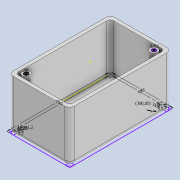
# Autodesk Inventor part: proper shit spodnji
Saved by Autodesk Inventor 2020 (Build 240168000, 168)
## iProperties
Created: 2020-08-03
Part Number: proper shit spodnji
Material: Generic
Document SubType Name: Modeling
Designer: borbu
Density: 1 g/cm^3
Appearance: Default
Author: borbu
Autodesk Inventor part; units mm, degrees
ref_plane "YZ Plane" through (0, 0, 0) normal (1, 0, 0) x (0, 1, 0)
ref_plane "XZ Plane" through (0, 0, 0) normal (0, 1, 0) x (-1, 0, 0)
ref_plane "XY Plane" through (0, 0, 0) normal (0, 0, 1) x (1, 0, 0)
sketch "Sketch1" plane through (0, 0, 0) normal (0, 1, 0) x (-1, 0, 0)
  line L0 (-22.5, 37.5) -> (22.5, 37.5)
  line L1 (22.5, 37.5) -> (22.5, -37.5)
  line L2 (22.5, -37.5) -> (-22.5, -37.5)
  line L3 (-22.5, -37.5) -> (-22.5, 37.5)
  line L4 (22.5, 37.5) -> (-22.5, -37.5) construction
  line L5 (-20, 35) -> (20, 35)
  line L6 (20, 35) -> (20, -35)
  line L7 (20, -35) -> (-20, -35)
  line L8 (-20, -35) -> (-20, 35)
  line L9 (20, 35) -> (-20, -35) construction
  line L10 (20, 35) -> (17.5, 35)
  line L11 (17.5, 35) -> (17.5, 32.5)
  line L12 (17.5, 32.5) -> (20, 32.5)
  line L13 (20, 32.5) -> (20, 35)
  arc A0 (20, 32.5) -> (17.5, 35) centre (17.5, 32.5) ccw
  line L14 (22.5, 37.5) -> (19, 37.5)
  line L15 (19, 37.5) -> (19, 34)
  line L16 (19, 34) -> (22.5, 34)
  line L17 (22.5, 34) -> (22.5, 37.5)
  line L18 (20, -35) -> (17.5, -35)
  line L19 (17.5, -35) -> (17.5, -32.5)
  line L20 (17.5, -32.5) -> (20, -32.5)
  line L21 (20, -32.5) -> (20, -35)
  line L22 (-20, -35) -> (-17.5, -35)
  line L23 (-17.5, -35) -> (-17.5, -32.5)
  line L24 (-17.5, -32.5) -> (-20, -32.5)
  line L25 (-20, -32.5) -> (-20, -35)
  line L26 (-20, 35) -> (-17.5, 35)
  line L27 (-17.5, 35) -> (-17.5, 32.5)
  line L28 (-17.5, 32.5) -> (-20, 32.5)
  line L29 (-20, 32.5) -> (-20, 35)
  arc A1 (-17.5, 35) -> (-20, 32.5) centre (-17.5, 32.5) ccw
  arc A2 (-20, -32.5) -> (-17.5, -35) centre (-17.5, -32.5) ccw
  arc A3 (17.5, -35) -> (20, -32.5) centre (17.5, -32.5) ccw
  arc A4 (22.5, 34) -> (19, 37.5) centre (19, 34) ccw
  line L30 (22.5, -37.5) -> (19, -37.5)
  line L31 (19, -37.5) -> (19, -34)
  line L32 (19, -34) -> (22.5, -34)
  line L33 (22.5, -34) -> (22.5, -37.5)
  line L34 (-22.5, -37.5) -> (-19, -37.5)
  line L35 (-19, -37.5) -> (-19, -34)
  line L36 (-19, -34) -> (-22.5, -34)
  line L37 (-22.5, -34) -> (-22.5, -37.5)
  line L38 (-22.5, 37.5) -> (-19, 37.5)
  line L39 (-19, 37.5) -> (-19, 34)
  line L40 (-19, 34) -> (-22.5, 34)
  line L41 (-22.5, 34) -> (-22.5, 37.5)
  arc A5 (-19, 37.5) -> (-22.5, 34) centre (-19, 34) ccw
  arc A6 (-22.5, -34) -> (-19, -37.5) centre (-19, -34) ccw
  arc A7 (19, -37.5) -> (22.5, -34) centre (19, -34) ccw
  point P0 (0, 0)
  point P1 (-19.5, -34)
  point P2 (-20, -34)
  dimension "d0" = 45
  dimension "d1" = 75
  dimension "d2" = 40
  dimension "d3" = 70
  dimension "d8" = 2.5
  dimension "d9" = 2.5
  constraints: 84 end point, 20 parallel, 16 point on circle, 10 horizontal, 10 perpendicular, 8 centre point, 8 coincident, 2 midpoint, 1 point on line
  measures "d0" distance of L1.end L2.end
  measures "d1" distance of L0.end L1.end
  measures "d2" distance of L6.end L7.end
  measures "d3" distance of L5.end L6.end
  measures "d8" distance of L12.end L11.end
  measures "d9" distance of L11.end L10.end
extrude "Extrusion3" add sketch "Sketch1" along normal blind 2.5 contours L0 L15 L5 L39 | L39 L5 L8 L40 A5 | L40 L8 L36 L3 | A4 L16 L6 L5 L15 | L39 A1 L40 L8 L5 | L5 A1 L39 | L36 L8 L7 L35 A6 | L40 A1 L8 | L15 A0 L5 | L5 L6 L16 A0 L15 | L1 L32 L6 L16 | L5 L11 L12 L6 L20 L19 L7 L23 L24 L8 L28 L27 | L27 L28 A1 L40 L39 | L39 L40 A1 | L36 A2 L35 L7 L8 | L35 L7 L31 L2 | A0 L15 L16 L12 L11 | A0 L16 L15 | A7 L31 L7 L6 L32 | L6 A0 L16 | L24 L23 A2 L35 L36 | L36 L35 A2 | L35 A2 L7 | L32 A3 L6 | L6 L7 L31 A3 L32 | L7 A3 L31 | A3 L32 L31 L19 L20 | A3 L31 L32
extrude "Extrusion4" add sketch "Sketch1" along normal blind 37.5 contours L0 L15 L5 L39 | L39 L5 L8 L40 A5 | L40 L8 L36 L3 | A4 L16 L6 L5 L15 | L39 A1 L40 L8 L5 | L5 A1 L39 | L36 L8 L7 L35 A6 | L40 A1 L8 | L15 A0 L5 | L5 L6 L16 A0 L15 | L1 L32 L6 L16 | L36 A2 L35 L7 L8 | L8 A2 L36 | L35 L7 L31 L2 | A7 L31 L7 L6 L32 | L6 A0 L16 | L35 A2 L7 | L32 A3 L6 | L6 L7 L31 A3 L32 | L7 A3 L31
fillet "Fillet1" radius 3 8 edges at (-21.4749, 0, 36.4749) (0, 0, 37.5) (21.4749, 0, 36.4749) (22.5, 0, 0) (21.4749, 0, -36.4749) (0, 0, -37.5) (-21.4749, 0, -36.4749) (-22.5, 0, 0)
sketch "Sketch2" plane through (0, 2.5, 0) normal (0, 1, 0) x (1, 0, 0)
  arc A0 (20, 32.5) -> (17.5, 35) centre (17.5, 32.5) ccw projected
  line L0 (17.5, 35) -> (17.5, 33.5)
  line L1 (20, -32.5) -> (20, 32.5) projected
  line L2 (20, 32.5) -> (18.5, 32.5)
  line L3 (18.5, 32.5) -> (17.5, 33.5)
  line L4 (18, 33) -> (16.0555, 31.0555)
  circle A1 centre (16.0555, 31.0555) radius 2.75
  line L5 (-20, 32.5) -> (-20, -32.5) projected
  line L6 (-20, -32.5) -> (-18.5, -32.5)
  line L7 (-17.5, -35) -> (17.5, -35) projected
  line L8 (-17.5, -35) -> (-17.5, -33.5)
  line L9 (-17.5, -33.5) -> (-18.5, -32.5)
  line L10 (-18, -33) -> (-16.0555, -31.0555)
  line L11 (-18, -33) -> (-15.25, -33) construction
  circle A2 centre (-16.0555, -31.0555) radius 2.75
  arc A3 (17.5812, 28.7675) -> (18.8055, 31.0555) centre (16.0555, 31.0555) ccw construction
  arc A4 (17.8504, 28.3639) -> (19.2906, 31.0555) centre (16.0555, 31.0555) ccw
  arc A5 (17.3121, 29.1712) -> (18.3203, 31.0555) centre (16.0555, 31.0555) ccw
  arc A6 (17.3121, 29.1712) -> (17.8504, 28.3639) centre (17.5812, 28.7675) ccw
  arc A7 (19.2906, 31.0555) -> (18.3203, 31.0555) centre (18.8055, 31.0555) ccw
  arc A8 (14.2605, 33.747) -> (12.8203, 31.0555) centre (16.0555, 31.0555) ccw
  arc A9 (12.8203, 31.0555) -> (13.7906, 31.0555) centre (13.3055, 31.0555) ccw
  arc A10 (14.7989, 32.9398) -> (14.2605, 33.747) centre (14.5297, 33.3434) ccw
  arc A11 (14.7989, 32.9398) -> (13.7906, 31.0555) centre (16.0555, 31.0555) ccw
  arc A12 (-14.2605, -33.747) -> (-12.8203, -31.0555) centre (-16.0555, -31.0555) ccw
  arc A13 (-14.7989, -32.9398) -> (-13.7906, -31.0555) centre (-16.0555, -31.0555) ccw
  arc A14 (-14.7989, -32.9398) -> (-14.2605, -33.747) centre (-14.5297, -33.3434) ccw
  arc A15 (-12.8203, -31.0555) -> (-13.7906, -31.0555) centre (-13.3055, -31.0555) ccw
  arc A16 (-17.8504, -28.3639) -> (-19.2906, -31.0555) centre (-16.0555, -31.0555) ccw
  arc A17 (-19.2906, -31.0555) -> (-18.3203, -31.0555) centre (-18.8055, -31.0555) ccw
  arc A18 (-17.3121, -29.1712) -> (-17.8504, -28.3639) centre (-17.5812, -28.7675) ccw
  arc A19 (-17.3121, -29.1712) -> (-18.3203, -31.0555) centre (-16.0555, -31.0555) ccw
  line L12 (-19.2843, -34.2843) -> (-16.7157, -31.7157) construction
  line L13 (-18.86, -34.7085) -> (-16.2915, -32.14)
  line L14 (-17.14, -31.2915) -> (-19.7085, -33.86)
  arc A20 (-19.7085, -33.86) -> (-18.86, -34.7085) centre (-19.2843, -34.2843) ccw
  arc A21 (-16.2915, -32.14) -> (-17.14, -31.2915) centre (-16.7157, -31.7157) ccw
  line L15 (16.5205, 31.5205) -> (19.4795, 34.4795) construction
  line L16 (16.9448, 31.0962) -> (19.9038, 34.0552)
  line L17 (19.0552, 34.9038) -> (16.0962, 31.9448)
  arc A22 (16.0962, 31.9448) -> (16.9448, 31.0962) centre (16.5205, 31.5205) ccw
  arc A23 (19.9038, 34.0552) -> (19.0552, 34.9038) centre (19.4795, 34.4795) ccw
  point P0 (0, 0)
  point P1 (18.3774, 32.5289)
  point P2 (17.5289, 33.3774)
  point P3 (14.9555, 33.5759)
  point P4 (13.3482, 30.5722)
  point P5 (17.1554, 28.535)
  point P6 (18.7627, 31.5387)
  point P7 (-18.3774, -32.5289)
  point P8 (-17.5289, -33.3774)
  point P9 (-14.9555, -33.5759)
  point P10 (-13.3482, -30.5722)
  point P11 (-17.1554, -28.535)
  point P12 (-18.7627, -31.5387)
  point P13 (18.7918, 34.6404)
  point P14 (19.6404, 33.7918)
  dimension "d32" = 5.5
  dimension "d29" = 1.5
  dimension "d30" = 1.5
  dimension "d31" = 2.75
  dimension "d33" = 1.5
  dimension "d34" = 1.5
  dimension "d35" = 2.75
  dimension "d36" = 45
  dimension "d37" = 5.5
  dimension "d40" = 360
  dimension "d44" = 1.2
  dimension "d45" = 1.2
  constraints: 42 point on circle, 34 end point, 22 centre point, 16 tangent, 4 midpoint, 3 coincident, 3 horizontal, 3 point on line, 2 parallel, 2 perpendicular, 2 vertical, 1 equal length, 27 other
  measures "d29" distance of L0.start L0.end
  measures "d30" distance of L1.end L2.end
  measures "d31" distance of L4.start L4.end
  measures "d33" distance of L5.end L6.end
  measures "d34" distance of L7.start L8.end
  measures "d35" distance of L10.start L10.end
  measures "d36" angle of L11 L10
  measures "d37" diameter of A2
  measures "d44" diameter of A21
  measures "d45" diameter of A23
extrude "Extrusion5" add sketch "Sketch2" along normal blind 35 contours A0 L17 A23 L16 | A1 L16 A22 L4 | L4 A22 L17 A1 | A1 A7 A5 A6 A9 A11 A10 L17 A22 L16 | A1 A6 A5 A7 | A10 A11 A9 A1 | A2 L14 A21 L10 | L10 A21 L13 A2 | L13 A21 L14 A2 A17 A19 A18 A15 A13 A14 | A14 A13 A15 A2 | A2 A18 A19 A17
extrude "Extrusion6" add sketch "Sketch2" along normal blind 10 contours A7 A4 A6 A1 | A1 A9 A8 A10 | A2 L14 A21 L10 | L10 A21 L13 A2 | L13 A21 L14 A2 A17 A19 A18 A15 A13 A14 | A14 A13 A15 A2 | A2 A15 A12 A14 | A17 A16 A18 A2 | A2 A18 A19 A17
sketch "Sketch3" plane through (0, 37.5, 0) normal (0, 1, 0) x (1, 0, 0)
  arc A0 (-13.3055, -31.0555) -> (-13.3055, -31.0555) centre (-16.0555, -31.0555) ccw projected
  circle A1 centre (-16.0555, -31.0555) radius 1.5
  circle A2 centre (-16.0555, -31.0555) radius 1.25
  circle A3 centre (16.0488, 31.0622) radius 1.5
  circle A4 centre (16.0488, 31.0622) radius 1.25
  point P0 (0, 0)
  dimension "d50" = 3
  dimension "d51" = 2.5
  dimension "d52" = 3
  dimension "d53" = 2.5
  constraints: 4 centre point, 3 coincident
  measures "d50" diameter of A1
  measures "d51" diameter of A2
  measures "d52" diameter of A3
  measures "d53" diameter of A4
extrude "Extrusion7" cut sketch "Sketch3" against normal blind 0.5 contours A1 | A3
extrude "Extrusion8" cut sketch "Sketch3" against normal blind 20 contours A2 | A4
extrude "Extrusion9" add sketch "Sketch2" along normal blind 32 contours L16 L3 L17 A0 | L16 A1 L3 | L3 A1 L17 | L13 A20 L14 L9 | L9 A2 L13 | L9 L14 A2
body "Solid2"
